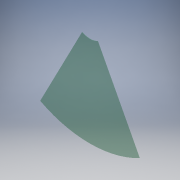
# Autodesk Inventor part: us-plane
Saved by Autodesk Inventor 2019 (Build 230136000, 136)
## iProperties
Created: 2020-05-04
Part Number: us-plane
Material: Leather, Dark Brown
Document SubType Name: Modeling
Designer: mx19
Density: 0.9 g/cm^3
Appearance: Clear - Green 1
Author: mx19
Autodesk Inventor part; units mm, degrees
ref_plane "YZ Plane" through (0, 0, 0) normal (1, 0, 0) x (0, 1, 0)
ref_plane "XZ Plane" through (0, 0, 0) normal (0, 1, 0) x (-1, 0, 0)
ref_plane "XY Plane" through (0, 0, 0) normal (0, 0, 1) x (1, 0, 0)
sketch "Sketch1" plane through (0, 0, 0) normal (0, 0, 1) x (1, 0, 0)
  arc A0 (-25.9041, -49.7613) -> (25.9041, -49.7613) centre (0, 0) ccw
  arc A1 (-164.4287, -315.8646) -> (164.4287, -315.8646) centre (0, 0) ccw
  line L0 (-25.9041, -49.7613) -> (-164.4287, -315.8646)
  line L1 (0, 0) -> (356.1, 0) construction
  line L2 (25.9041, -49.7613) -> (164.4287, -315.8646)
  line L3 (0, 0) -> (356.1, 0) construction
  dimension "d0" = 112.2
  dimension "d1" = 712.2
  dimension "d2" = 117.5
  dimension "d3" = 62.5
  constraints: 8 end point, 4 point on circle, 2 centre point, 2 coincident, 2 horizontal
  measures "d0" diameter of A0
  measures "d1" diameter of A1
  measures "d2" angle of L0 L1
  measures "d3" angle of L2 L3
extrude "Extrusion1" add sketch "Sketch1" along normal blind 1
body "Solid1"
